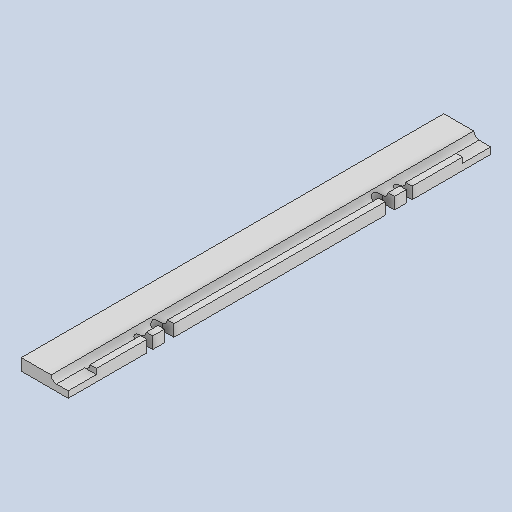
# Autodesk Inventor part: test2
Saved by Autodesk Inventor 2025 (Build 290162000, 162)
## iProperties
Created: 2025-04-20
Part Number: test2
Material: Generic
Document SubType Name: Sheet Metal
Designer: Pravoslav
Density: 1 g/cm^3
Sheet Metal Rule: Default_mm
Appearance: Default
Author: Pravoslav
Autodesk Inventor part; units mm, degrees
ref_plane "YZ Plane" through (0, 0, 0) normal (1, 0, 0) x (0, 1, 0)
ref_plane "XZ Plane" through (0, 0, 0) normal (0, 1, 0) x (-1, 0, 0)
ref_plane "XY Plane" through (0, 0, 0) normal (0, 0, 1) x (1, 0, 0)
sketch "Sketch1" plane through (0, 0, 0) normal (0, 1, 0) x (-1, 0, 0)
  line L0 (5, 90) -> (-5, 90)
  line L1 (-5, 90) -> (-5, -90)
  line L2 (-5, -90) -> (5, -90)
  line L3 (5, -90) -> (5, 90)
  line L4 (5, 90) -> (-5, -90) construction
  line L5 (-5, 90) -> (5, -90) construction
  point P0 (0, 0)
  dimension "d0" = 10
  dimension "d1" = 180
  constraints: 12 end point, 2 midpoint, 2 parallel, 1 horizontal, 1 perpendicular
  measures "d0" distance of L2.end L1.end
  measures "d1" distance between parallel lines of L2 L0
extrude "Extrusion1" add sketch "Sketch1" along normal blind 5
sketch "Sketch2" plane through (0, 5, 0) normal (0, 1, 0) x (1, 0, 0)
  line L0 (-5, 90) -> (-5, -90) projected
  line L1 (-5, -45) -> (5.6996, -45)
  line L2 (-5, 45) -> (5, 45)
  line L3 (5, -90) -> (5, 90) projected
  line L4 (-5, -49) -> (5, -49)
  line L5 (-5, 49) -> (5, 49)
  line L6 (-5, -54) -> (5, -54)
  line L7 (-5, 54) -> (5, 54)
  line L8 (-5, 56.5) -> (5, 56.5)
  line L9 (-5, -56.5) -> (5, -56.5)
  line L10 (-5, -56.5) -> (5, -56.5)
  line L11 (5, -56.5) -> (5, -54)
  line L12 (5, -54) -> (-5, -54)
  line L13 (-5, -54) -> (-5, -56.5)
  line L14 (-5, -49) -> (5, -49)
  line L15 (5, -49) -> (5, -45)
  line L16 (5, -45) -> (-5, -45)
  line L17 (-5, -45) -> (-5, -49)
  line L18 (-4.366, 45) -> (5, 45)
  line L19 (5, 45) -> (5, 49)
  line L20 (5, 49) -> (-4.366, 49)
  line L21 (-4.366, 49) -> (-4.366, 45)
  line L22 (-5, 54) -> (5, 54)
  line L23 (5, 54) -> (5, 56.5)
  line L24 (5, 56.5) -> (-5, 56.5)
  line L25 (-5, 56.5) -> (-5, 54)
  circle A0 centre (0, -55.25) radius 1.25
  circle A1 centre (0, -47) radius 2
  circle A2 centre (0, 47) radius 2.025
  circle A3 centre (0, 55.25) radius 1.25
  point P0 (0, 0)
  point P1 (-0.317, 49)
  point P2 (-0.317, 45)
  point P3 (0.317, 45)
  point P4 (0.317, 49)
  dimension "d4" = 90
  dimension "d5" = 45
  dimension "d6" = 4
  dimension "d7" = 4
  dimension "d8" = 5
  dimension "d9" = 5
  dimension "d10" = 2.5
  dimension "d11" = 2.5
  constraints: 48 end point, 12 horizontal, 8 parallel, 4 centre point, 4 perpendicular, 3 tangent, 2 point on line, 18 other
  measures "d4" distance between parallel lines of L2 L1
  measures "d5" distance from line of L2 point (0, 0)
  measures "d6" distance between parallel lines of L1 L4
  measures "d7" distance between parallel lines of L5 L2
  measures "d8" distance between parallel lines of L6 L4
  measures "d9" distance between parallel lines of L5 L7
  measures "d10" distance between parallel lines of L6 L9
  measures "d11" distance between parallel lines of L7 L8
sketch "Sketch3" plane through (5, 0, 90) normal (1, 0, 0) x (0, 0, -1)
  line L0 (33.5, 5) -> (36, 5) projected
  line L1 (41, 5) -> (45, 5) projected
  line L2 (0, 5) -> (180, 5) projected
  line L3 (0, 0) -> (180, 0) projected
  line L4 (33.5, 5) -> (36, 5)
  line L5 (36, 5) -> (36, 0)
  line L6 (36, 0) -> (33.5, 0)
  line L7 (33.5, 0) -> (33.5, 5)
  line L8 (41, 5) -> (45, 5)
  line L9 (45, 5) -> (45, 0)
  line L10 (45, 0) -> (41, 0)
  line L11 (41, 0) -> (41, 5)
  line L12 (180, 0) -> (0, 0) projected
  line L13 (135, 5) -> (139, 5)
  line L14 (139, 5) -> (139, 0)
  line L15 (139, 0) -> (135, 0)
  line L16 (135, 0) -> (135, 5)
  line L17 (144, 5) -> (146.5, 5)
  line L18 (146.5, 5) -> (146.5, 0)
  line L19 (146.5, 0) -> (144, 0)
  line L20 (144, 0) -> (144, 5)
  point P0 (90, 0)
  point P1 (135, 2.5)
  point P2 (45, 2.5)
  point P3 (90, 0)
  point P4 (144, 2.5)
  point P5 (36, 2.5)
  point P6 (41, 2.5)
  dimension "d12" = 4
  dimension "d13" = 2.5
  dimension "d14" = 90
  dimension "d15" = 45
  dimension "d16" = 5
  dimension "d17" = 5
  constraints: 32 end point, 8 parallel, 6 midpoint, 4 horizontal, 4 perpendicular, 4 point on line, 3 other
  measures "d12" distance of L14.end L15.end
  measures "d13" distance of L18.end L19.end
  measures "d14" distance of point (135, 2.5) point (45, 2.5)
  measures "d15" horizontal distance of point (90, 0) point (135, 2.5)
  measures "d16" distance from line of point (144, 2.5) L14
  measures "d17" distance of point (36, 2.5) point (41, 2.5)
extrude "Extrusion2" cut sketch "Sketch2" against normal through all contours A3 | L5 A2 L2 | A1 | A0
extrude "Extrusion3" cut sketch "Sketch3" against normal up to next contours L0 L5 L3 L7 | L2 L18 L3 L20
extrude "Extrusion4" cut sketch "Sketch3" against normal up to next contours L1 L9 L3 L11 | L2 L14 L3 L16
sketch "Sketch4" plane through (5, 0, -90) normal (0, 0, -1) x (-1, 0, 0)
  line L0 (5, 5) -> (6.25, 5) projected
  circle A0 centre (5, 5) radius 2.25
  point P0 (5, 0)
  dimension "d24" = 4.5
  constraints: 1 centre point
  measures "d24" diameter of A0
extrude "Extrusion5" cut sketch "Sketch4" against normal through all
sketch "Sketch5" plane through (5, 0, -90) normal (0, 0, -1) x (-1, 0, 0)
  line L0 (0, 0) -> (0, 5) projected
  line L1 (10, 5) -> (10, 3)
  line L2 (0, 3) -> (0, 5)
  line L3 (10, 5) -> (10, 3)
  arc A0 (2.75, 5) -> (5, 2.75) centre (5, 5) ccw projected
  line L4 (2.75, 5) -> (0, 5) projected
  line L5 (5, 2.75) -> (0, 2.75)
  line L6 (0, 2.75) -> (0, 5)
  line L7 (0, 5) -> (5, 5)
  line L8 (5, 5) -> (5, 2.75)
  point P0 (5, 0)
  point P1 (0, 2.75)
  dimension "d27" = 2
  constraints: 14 end point, 3 parallel, 1 horizontal, 1 perpendicular
  measures "d27" distance of L1.start L1.end
extrude "Extrusion6" cut sketch "Sketch5" against normal blind 12 contours L0 L4 A0 L5
mirror "Mirror2" about plane through (0, 0, 0) normal (0, 0, 1) of "Extrusion6"
sketch "Sketch6" plane through (-5, 0, -90) normal (-1, 0, 0) x (0, 0, 1)
  line L0 (0, 5) -> (180, 5) projected
  line L1 (0, 5) -> (180, 5)
  line L2 (180, 5) -> (180, 0)
  line L3 (180, 0) -> (0, 0)
  line L4 (0, 0) -> (0, 5)
  line L5 (0, 5) -> (180, 5)
  line L6 (180, 5) -> (180, 0)
  line L7 (180, 0) -> (0, 0)
  line L8 (0, 0) -> (0, 5)
  point P0 (90, 0)
  constraints: 16 end point, 4 parallel, 2 horizontal, 2 perpendicular
extrude "Extrusion7" add sketch "Sketch6" along normal blind 10
equation "\"BendRadius\" = Thickness"
equation "\"BendReliefWidth\" = Thickness"
equation "\"BendReliefDepth\" = 0.5 * Thickness"
equation "\"CornerReliefSize\" = 4 * Thickness"
equation "\"MinimumRemnant\" = 2 * Thickness"
equation "\"TransitionRadius\" = BendRadius"
equation "\"JacobiRadiusSize\" = BendRadius"
equation "\"GapSize\" = Thickness"
equation "\"Thickness\" = 0.5"
body "Solid1"
